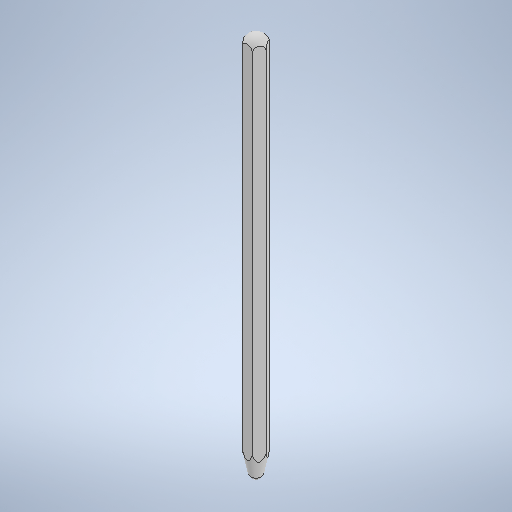
# Autodesk Inventor part: stylus_pen
Saved by Autodesk Inventor 2025.1 (Build 291241000, 241)
## iProperties
Created: 2024-08-22
Part Number: stylus_pen
Material: Generic
Document SubType Name: Modeling
Designer: pedro
Density: 1 g/cm^3
Appearance: Default
Author: pedro
Autodesk Inventor part; units mm, degrees
ref_plane "YZ Plane" through (0, 0, 0) normal (1, 0, 0) x (0, 1, 0)
ref_plane "XZ Plane" through (0, 0, 0) normal (0, 1, 0) x (-1, 0, 0)
ref_plane "XY Plane" through (0, 0, 0) normal (0, 0, 1) x (1, 0, 0)
sketch "Sketch1" plane through (0, 0, 0) normal (0, 1, 0) x (-1, 0, 0)
  line L0 (-4.5, 0) -> (-2.25, 3.8971)
  line L1 (-2.25, 3.8971) -> (2.25, 3.8971)
  line L2 (2.25, 3.8971) -> (4.5, 0)
  line L3 (4.5, 0) -> (2.25, -3.8971)
  line L4 (2.25, -3.8971) -> (-2.25, -3.8971)
  line L5 (-2.25, -3.8971) -> (-4.5, 0)
  point P0 (0, 0)
  point P1 (0, 0)
  dimension "d1" = 9
  constraints: 12 end point, 1 coincident, 13 other
  measures "d1" distance of L0.start L2.end
extrude "Extrusion1" add sketch "Sketch1" along normal blind 155
sketch "Sketch2" plane through (0, 0, 0) normal (0, 0, 1) x (1, 0, 0)
  line L0 (2.25, 155) -> (-2.25, 155) projected
  line L1 (2.25, 155) -> (4.5, 155) projected
  arc A0 (4.5, 155) -> (0, 159.5) centre (0, 155) ccw
  line L2 (0, 155) -> (0, 159.5)
  line L3 (0, 155) -> (4.5, 155)
  point P0 (0, 0)
  constraints: 4 end point, 2 point on circle, 1 centre point, 1 midpoint, 1 perpendicular, 1 vertical
revolve "Revolution1" add sketch "Sketch2" angle 360 about axis through (0, 155, 0) along (0, 1, 0)
sketch "Sketch3" plane through (0, 0, 0) normal (0, -1, 0) x (1, 0, 0)
  line L0 (2.25, -3.8971) -> (-2.25, -3.8971) projected
  arc A0 (-4.5, 0) -> (-2.25, -3.8971) centre (0, 0) ccw projected
  line L1 (2.25, -3.8971) -> (-2.25, -3.8971)
  line L2 (-2.25, -3.8971) -> (-4.5, 0) projected
  line L3 (-2.25, -3.8971) -> (-4.5, 0)
  arc A1 (-2.25, 3.8971) -> (-4.5, 0) centre (0, 0) ccw projected
  line L4 (-4.5, 0) -> (-2.25, 3.8971)
  arc A2 (2.25, 3.8971) -> (-2.25, 3.8971) centre (0, 0) ccw projected
  line L5 (-2.25, 3.8971) -> (2.25, 3.8971)
  line L6 (2.25, 3.8971) -> (4.5, 0)
  line L7 (4.5, 0) -> (2.25, -3.8971)
  point P0 (0, 0)
  constraints: 12 end point, 4 equal length, 1 horizontal
extrude "Extrusion2" cut sketch "Sketch3" along normal mid plane 400 contours L0 L2 L4 L5 L6 L7 keep common part
sketch "Sketch4" plane through (0, 0, 0) normal (0, 0, 1) x (1, 0, 0)
  line L0 (-4.5, 0) -> (-4.5, 155) projected
  line L1 (0, 0) -> (-4.5, 0)
  line L2 (0, 0) -> (0, -10)
  line L3 (0, -10) -> (-2.5, -10)
  line L4 (-4.5, 0) -> (-2.5, -10)
  point P0 (-4.5, 100)
  dimension "d7" = 10
  dimension "d9" = 2.5
  constraints: 8 end point, 1 horizontal, 1 perpendicular, 1 vertical
  measures "d7" distance of L2.end L1.start
  measures "d9" distance from line of L2 L3.end
revolve "Revolution2" add sketch "Sketch4" angle 360 about axis through (0, 0, 0) along (0, -1, 0)
thicken "Thicken1" operation cut thickness 5 both sides no extend neighbours no toward (0, -1, 0) faces at (-0.4635, 0, 4.0247)
thicken "Thicken2" operation cut thickness 5 both sides no extend neighbours no toward (0, -1, 0) faces at (-3.2537, 0, 2.4138)
thicken "Thicken3" operation cut thickness 5 both sides no extend neighbours no toward (0, -1, 0) faces at (-3.7172, 0, -1.6109)
thicken "Thicken4" operation cut thickness 5 both sides no extend neighbours no toward (0, -1, 0) faces at (3.4635, 0, 2.1807)
thicken "Thicken5" operation cut thickness 5 both sides no extend neighbours no toward (0, -1, 0) faces at (3.7172, 0, -1.6109)
thicken "Thicken6" operation cut thickness 5 both sides no extend neighbours no toward (0, -1, 0) faces at (0.1568, 0, -4.0899)
sketch "Sketch5" plane through (0, 0, 0) normal (0, 0, 1) x (1, 0, 0)
  line L0 (-2.5, -10) -> (2.5, -10) projected
  arc A0 (2, -10) -> (0, -12) centre (0, -10) ccw
  line L1 (0, -10) -> (0, -12)
  line L2 (2.5, -10) -> (2, -10)
  line L3 (-2, -10) -> (-2.5, -10)
  line L4 (0, -10) -> (-2, -10)
  point P0 (0, 0)
  point P1 (-2, -10)
  dimension "d23" = 4
  constraints: 8 end point, 3 horizontal, 3 point on circle, 1 centre point, 1 vertical
  measures "d23" diameter of A0
revolve "Revolution3" add sketch "Sketch5" angle 360 about axis through (0, -10, 0) along (0, -1, 0) contours L0 L1 A0
body "Solid1"
